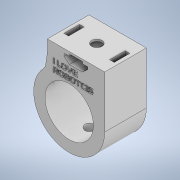
# Autodesk Inventor part: MotorBearingHolder
Saved by Autodesk Inventor 2020 (Build 240168000, 168)
## iProperties
Created: 2020-01-14
Part Number: MotorBearingHolder
Material: Generic
Document SubType Name: Modeling
Designer: yukin
Density: 1 g/cm^3
Appearance: Default
Author: yukin
Autodesk Inventor part; units mm, degrees
note: some values were not read from the file. Chosen so that the rebuilt part matches the saved one: direction of "Emboss1".
ref_plane "YZ Plane" through (0, 0, 0) normal (1, 0, 0) x (0, 1, 0)
sketch "Sketch1" plane through (0, 0, 0) normal (0, 0, 1) x (1, 0, 0)
  line L0 (-13.97, -12.7) -> (13.97, -12.7)
  line L1 (13.97, -12.7) -> (13.97, 12.7)
  line L2 (13.97, 12.7) -> (-13.97, 12.7)
  line L3 (-13.97, 12.7) -> (-13.97, -12.7)
  line L4 (-13.97, -12.7) -> (13.97, 12.7) construction
  line L5 (13.97, -12.7) -> (-13.97, 12.7) construction
  arc A0 (-13.97, -12.7) -> (13.97, -12.7) centre (0, -12.7) ccw
  circle A1 centre (-3.3455, -12.7) radius 11.811
  line L6 (0, -12.7) -> (-13.97, -12.7)
  line L7 (0, -12.7) -> (-6.985, -12.7)
  circle A2 centre (-3.3455, -12.7) radius 17.3155
  arc A3 (-20.6609, -12.7) -> (-13.97, 12.7) centre (-56.001, 10.1906) ccw
  point P0 (0, 0)
  point P1 (-15.1565, -0.038)
  dimension "d0" = 27.94
  dimension "d1" = 25.4
  dimension "d2" = 23.622
  constraints: 16 end point, 6 point on circle, 4 centre point, 3 midpoint, 2 parallel, 2 tangent, 1 coincident, 1 horizontal, 1 perpendicular
  measures "d0" distance of L1.end L2.end
  measures "d1" distance of L0.end L1.end
  measures "d2" diameter of A1
sketch "Sketch5" plane through (0, 0, 0) normal (0, 0, 1) x (1, 0, 0)
  line L0 (0, 12.7) -> (0, 6.35)
  line L1 (0, 12.7) -> (0, 9.525)
  line L2 (5.715, 7.3025) -> (-5.715, 7.3025)
  line L3 (-5.715, 7.3025) -> (-5.715, 11.7475)
  line L4 (-5.715, 11.7475) -> (5.715, 11.7475)
  line L5 (5.715, 11.7475) -> (5.715, 7.3025)
  line L6 (5.715, 7.3025) -> (-5.715, 11.7475) construction
  line L7 (-5.715, 7.3025) -> (5.715, 11.7475) construction
  line L8 (5.715, 11.7475) -> (3.175, 11.7475)
  line L9 (3.175, 11.7475) -> (3.175, 10.7597)
  line L10 (3.175, 10.7597) -> (5.715, 10.7597)
  line L11 (5.715, 10.7597) -> (5.715, 11.7475)
  line L12 (-5.715, 11.7475) -> (-3.2581, 11.7475)
  line L13 (-3.2581, 11.7475) -> (-3.2581, 10.792)
  line L14 (-3.2581, 10.792) -> (-5.715, 10.792)
  line L15 (-5.715, 10.792) -> (-5.715, 11.7475)
  line L16 (5.715, 9.525) -> (3.175, 7.3025)
  line L17 (-5.715, 9.525) -> (-3.175, 7.3025)
  point P0 (0, 0)
  point P1 (5.715, 10.7597)
  point P2 (-3.2581, 11.7475)
  point P3 (-5.715, 10.792)
  dimension "d5" = 4.445
  dimension "d6" = 11.43
  dimension "d7" = 2.54
  constraints: 36 end point, 6 parallel, 5 midpoint, 4 point on line, 3 horizontal, 3 perpendicular
  measures "d5" distance of L2.end L3.end
  measures "d6" distance of L2.start L2.end
  measures "d7" distance of L10.end L9.end
ref_plane "Work Plane4" through (-13.97, 12.7, 0) normal (0, 1, 0) x (1, 0, 0)
sketch "Sketch6" plane through (-13.97, 12.7, 0) normal (0, 1, 0) x (1, 0, 0)
  circle A0 centre (13.97, -10.16) radius 2.54
  dimension "d19" = 5.08
  constraints: 1 centre point
  measures "d19" diameter of A0
extrude "Extrusion7" add sketch "Sketch1" along normal blind 20.32 contours A1 A0 A2 A3 L3 | L3 A2 L0 A1 | A1 L0 A0 | A2 A3 L3 | L3 A3 L2 L1 A2 | A3 A2 picked at (12.0052, -13.7923)
extrude "Extrusion8" cut sketch "Sketch5" along normal blind 20.32 contours L4 L9 L10 L5 L16 L2 L0 | L0 L2 L17 L3 L14 L13 L4
extrude "Extrusion9" cut sketch "Sketch6" against normal blind 15.24
fillet "Fillet1" radius 3.175 1 edges at (-15.1565, -0.038, 10.16)
sketch "Sketch10" plane through (-13.97, 12.7, 0) normal (0, 1, 0) x (1, 0, 0)
  line L0 (13.97, 0) -> (13.97, -20.32)
  line L1 (0.0748, -20.32) -> (0.0748, 0) projected
  line L2 (0.0748, -10.16) -> (27.94, -10.16)
  line L3 (27.94, 0) -> (27.94, -20.32) projected
  line L4 (3.9773, -13.97) -> (1.6913, -13.97)
  line L5 (1.6913, -13.97) -> (1.6913, -6.35)
  line L6 (1.6913, -6.35) -> (3.9773, -6.35)
  line L7 (3.9773, -6.35) -> (3.9773, -13.97)
  line L8 (3.9773, -13.97) -> (1.6913, -6.35) construction
  line L9 (1.6913, -13.97) -> (3.9773, -6.35) construction
  line L10 (23.9627, -13.97) -> (26.2487, -13.97)
  line L11 (26.2487, -13.97) -> (26.2487, -6.35)
  line L12 (26.2487, -6.35) -> (23.9627, -6.35)
  line L13 (23.9627, -6.35) -> (23.9627, -13.97)
  point P0 (2.8343, -10.16)
  dimension "d32" = 2.286
  dimension "d33" = 7.62
  constraints: 24 end point, 4 midpoint, 4 symmetric about line, 2 parallel, 1 horizontal, 1 perpendicular, 1 point on line
  measures "d32" distance of L5.end L6.end
  measures "d33" distance of L6.end L4.start
extrude "Extrusion10" cut sketch "Sketch10" against normal blind 2.54
ref_plane "Work Plane5" through (-3.3455, -30.0155, 0) normal (0, 1, 0) x (-1, 0, 0)
sketch "Sketch11" plane through (-3.3455, -30.0155, 0) normal (0, 1, 0) x (-1, 0, 0)
  line L0 (-0.1705, 0) -> (-0.1705, 20.32) projected
  circle A0 centre (-0.1705, 10.16) radius 2.54
  point P0 (-3.3455, 0)
  dimension "d36" = 5.08
  constraints: 1 centre point, 1 midpoint
  measures "d36" diameter of A0
extrude "Extrusion11" cut sketch "Sketch11" along normal blind 15.24
sketch "Sketch12" plane through (0, 0, 20.32) normal (0, 0, 1) x (1, 0, 0)
  line L0 (-11.2307, 6.2995) -> (3.6868, 6.2995) construction
  line L1 (3.6868, 6.2995) -> (3.6868, 2.8789) construction
  line L2 (3.6868, 2.8789) -> (-11.2307, 2.8789) construction
  line L3 (-11.2307, 2.8789) -> (-11.2307, 6.2995) construction
  spline S0 degree 2 poles (-10.4241, 3.896) (-10.4282, 3.8288) (-10.526, 3.733) (-10.5972, 3.7371) knots 0 0 0 1 2 2 2
  line L4 (-10.5972, 3.7371) -> (-10.8702, 3.7534)
  spline S1 degree 2 poles (-10.8702, 3.7534) (-10.9374, 3.7575) (-11.0352, 3.8654) (-11.0352, 3.9327) knots 0 0 0 1 2 2 2
  line L5 (-11.0352, 3.9327) -> (-11.0698, 6.1345)
  spline S2 degree 2 poles (-11.0698, 6.1345) (-11.0698, 6.2058) (-10.968, 6.3016) (-10.8946, 6.2934) knots 0 0 0 1 2 2 2
  line L6 (-10.8946, 6.2934) -> (-10.5606, 6.2649)
  spline S3 degree 2 poles (-10.5606, 6.2649) (-10.4954, 6.2588) (-10.4017, 6.1549) (-10.4017, 6.1284) knots 0 0 0 1 2 2 2
  line L7 (-10.4017, 6.1284) -> (-10.4241, 3.896)
  spline S4 degree 2 poles (-9.1898, 6.0999) (-9.1898, 6.1671) (-9.0859, 6.2608) (-9.0146, 6.2547) knots 0 0 0 1 2 2 2
  line L8 (-9.0146, 6.2547) -> (-8.6805, 6.2242)
  spline S5 degree 2 poles (-8.6805, 6.2242) (-8.6194, 6.216) (-8.5196, 6.1182) (-8.5196, 6.0775) knots 0 0 0 1 2 2 2
  line L9 (-8.5196, 6.0775) -> (-8.5583, 4.3767)
  spline S6 degree 2 poles (-8.5583, 4.3767) (-8.5583, 4.3197) (-8.5135, 4.281) (-8.485, 4.283) knots 0 0 0 1 2 2 2
  line L10 (-8.485, 4.283) -> (-7.3912, 4.3217)
  spline S7 degree 2 poles (-7.3912, 4.3217) (-7.3403, 4.3217) (-7.2995, 4.281) knots 0 0 0 1 1 1
  spline S8 degree 2 poles (-7.2995, 4.281) (-7.2466, 4.2423) (-7.2466, 4.1791) knots 0 0 0 1 1 1
  line L11 (-7.2466, 4.1791) -> (-7.2812, 3.8899)
  spline S9 degree 2 poles (-7.2812, 3.8899) (-7.2771, 3.8288) (-7.3627, 3.7371) (-7.4278, 3.7371) knots 0 0 0 1 2 2 2
  line L12 (-7.4278, 3.7371) -> (-8.705, 3.7371)
  spline S10 degree 2 poles (-8.705, 3.7371) (-8.8027, 3.7371) (-8.9718, 3.8105) (-9.0961, 3.9347) (-9.1694, 4.1038) (-9.1694, 4.2015) knots 0 0 0 1 2 3 4 4 4
  line L13 (-9.1694, 4.2015) -> (-9.1898, 6.0999)
  spline S11 degree 2 poles (-4.6719, 5.6701) (-4.6577, 5.55) (-4.6353, 5.2383) (-4.6312, 4.9165) (-4.6434, 4.6008) (-4.6577, 4.4724) knots 0 0 0 1 2 3 4 4 4
  spline S12 degree 2 poles (-4.6577, 4.4724) (-4.6882, 4.1588) (-5.0039, 3.8288) (-5.3197, 3.7819) knots 0 0 0 1 2 2 2
  spline S13 degree 2 poles (-5.3197, 3.7819) (-5.4134, 3.7677) (-5.7006, 3.7493) (-6.0122, 3.7453) (-6.3218, 3.7555) (-6.44, 3.7677) knots 0 0 0 1 2 3 4 4 4
  spline S14 degree 2 poles (-6.44, 3.7677) (-6.6885, 3.786) (-7.051, 4.1241) (-7.0897, 4.395) knots 0 0 0 1 2 2 2
  spline S15 degree 2 poles (-7.0897, 4.395) (-7.1121, 4.5437) (-7.1305, 4.9002) (-7.1345, 5.2485) (-7.1203, 5.5683) (-7.104, 5.6783) knots 0 0 0 1 2 3 4 4 4
  spline S16 degree 2 poles (-7.104, 5.6783) (-7.0816, 5.8738) (-6.7883, 6.1569) (-6.5561, 6.1895) knots 0 0 0 1 2 2 2
  spline S17 degree 2 poles (-6.5561, 6.1895) (-6.4461, 6.1997) (-6.1141, 6.2262) (-5.7515, 6.2466) (-5.3971, 6.2527) (-5.2687, 6.2486) knots 0 0 0 1 2 3 4 4 4
  spline S18 degree 2 poles (-5.2687, 6.2486) (-4.9856, 6.2364) (-4.7045, 5.941) (-4.6719, 5.6701) knots 0 0 0 1 2 2 2
  spline S19 degree 2 poles (-5.34, 5.717) (-5.45, 5.7292) (-5.7332, 5.7333) (-6.0285, 5.7292) (-6.2933, 5.7068) (-6.387, 5.6925) knots 0 0 0 1 2 3 4 4 4
  spline S20 degree 2 poles (-6.387, 5.6925) (-6.4359, 5.6803) (-6.5051, 5.5988) (-6.5072, 5.5377) knots 0 0 0 1 2 2 2
  spline S21 degree 2 poles (-6.5072, 5.5377) (-6.5133, 5.44) (-6.5133, 5.1263) (-6.5031, 4.835) (-6.4848, 4.5478) (-6.4664, 4.4419) knots 0 0 0 1 2 3 4 4 4
  spline S22 degree 2 poles (-6.4664, 4.4419) (-6.4562, 4.3584) (-6.3666, 4.2749) (-6.2974, 4.2647) knots 0 0 0 1 2 2 2
  spline S23 degree 2 poles (-6.2974, 4.2647) (-6.2098, 4.2545) (-5.9531, 4.2463) (-5.6904, 4.2545) (-5.45, 4.2789) (-5.3665, 4.3013) knots 0 0 0 1 2 3 4 4 4
  spline S24 degree 2 poles (-5.3665, 4.3013) (-5.2952, 4.3197) (-5.2199, 4.4134) (-5.2137, 4.4724) knots 0 0 0 1 2 2 2
  spline S25 degree 2 poles (-5.2137, 4.4724) (-5.2015, 4.6048) (-5.1873, 4.9022) (-5.1832, 5.1976) (-5.1913, 5.4685) (-5.1995, 5.5683) knots 0 0 0 1 2 3 4 4 4
  spline S26 degree 2 poles (-5.1995, 5.5683) (-5.2056, 5.6274) (-5.283, 5.7109) (-5.34, 5.717) knots 0 0 0 1 2 2 2
  spline S27 degree 2 poles (-2.3417, 6.1794) (-2.3112, 6.2343) (-2.1829, 6.2792) (-2.1238, 6.2506) knots 0 0 0 1 2 2 2
  line L14 (-2.1238, 6.2506) -> (-1.8508, 6.1284)
  spline S28 degree 2 poles (-1.8508, 6.1284) (-1.7857, 6.102) (-1.7531, 5.9818) (-1.7714, 5.939) knots 0 0 0 1 2 2 2
  line L15 (-1.7714, 5.939) -> (-2.6147, 4.0264)
  spline S29 degree 2 poles (-2.6147, 4.0264) (-2.6839, 3.8797) (-2.9589, 3.733) (-3.2563, 3.733) (-3.5252, 3.8777) (-3.5965, 4.0223) knots 0 0 0 1 2 3 4 4 4
  line L16 (-3.5965, 4.0223) -> (-4.4377, 5.939)
  spline S30 degree 2 poles (-4.4377, 5.939) (-4.456, 5.9818) (-4.4275, 6.0999) (-4.3521, 6.1325) knots 0 0 0 1 2 2 2
  line L17 (-4.3521, 6.1325) -> (-4.0894, 6.2486)
  spline S31 degree 2 poles (-4.0894, 6.2486) (-4.0324, 6.2792) (-3.8979, 6.2343) (-3.8714, 6.1753) knots 0 0 0 1 2 2 2
  line L18 (-3.8714, 6.1753) -> (-3.1259, 4.3869)
  spline S32 degree 2 poles (-3.1259, 4.3869) (-3.1219, 4.3787) (-3.0893, 4.3787) (-3.0832, 4.3869) knots 0 0 0 1 2 2 2
  line L19 (-3.0832, 4.3869) -> (-2.3417, 6.1794)
  line L20 (-0.9689, 4.7433) -> (-0.9648, 4.393)
  spline S33 degree 2 poles (-0.9648, 4.393) (-0.9628, 4.3604) (-0.922, 4.3197) (-0.8935, 4.3176) knots 0 0 0 1 2 2 2
  line L21 (-0.8935, 4.3176) -> (0.6443, 4.2463)
  spline S34 degree 2 poles (0.6443, 4.2463) (0.7177, 4.2463) (0.7645, 4.2076) knots 0 0 0 1 1 1
  spline S35 degree 2 poles (0.7645, 4.2076) (0.8175, 4.1649) (0.8175, 4.118) knots 0 0 0 1 1 1
  line L22 (0.8175, 4.118) -> (0.8093, 3.9449)
  spline S36 degree 2 poles (0.8093, 3.9449) (0.8093, 3.8736) (0.7279, 3.7819) (0.6586, 3.7819) knots 0 0 0 1 2 2 2
  line L23 (0.6586, 3.7819) -> (-1.087, 3.7636)
  spline S37 degree 2 poles (-1.087, 3.7636) (-1.2866, 3.7636) (-1.4292, 3.894) knots 0 0 0 1 1 1
  spline S38 degree 2 poles (-1.4292, 3.894) (-1.5718, 4.0365) (-1.5718, 4.2362) knots 0 0 0 1 1 1
  line L24 (-1.5718, 4.2362) -> (-1.5494, 5.7822)
  spline S39 degree 2 poles (-1.5494, 5.7822) (-1.5494, 5.8759) (-1.4801, 6.0429) (-1.364, 6.1631) (-1.197, 6.2425) (-1.0646, 6.2425) knots 0 0 0 1 2 3 4 4 4
  line L25 (-1.0646, 6.2425) -> (0.5975, 6.269)
  spline S40 degree 2 poles (0.5975, 6.269) (0.6647, 6.2751) (0.7116, 6.2282) knots 0 0 0 1 1 1
  spline S41 degree 2 poles (0.7116, 6.2282) (0.7523, 6.1956) (0.7625, 6.1325) knots 0 0 0 1 1 1
  line L26 (0.7625, 6.1325) -> (0.7706, 5.8535)
  spline S42 degree 2 poles (0.7706, 5.8535) (0.7747, 5.7903) (0.6892, 5.6986) (0.6219, 5.6986) knots 0 0 0 1 2 2 2
  line L27 (0.6219, 5.6986) -> (-0.9118, 5.7598)
  spline S43 degree 2 poles (-0.9118, 5.7598) (-0.9404, 5.7598) (-0.9607, 5.7353) knots 0 0 0 1 1 1
  spline S44 degree 2 poles (-0.9607, 5.7353) (-0.9811, 5.7211) (-0.9811, 5.6538) knots 0 0 0 1 1 1
  line L28 (-0.9811, 5.6538) -> (-0.977, 5.2628)
  line L29 (-0.977, 5.2628) -> (0.4529, 5.334)
  spline S45 degree 2 poles (0.4529, 5.334) (0.5201, 5.3422) (0.5649, 5.2953) knots 0 0 0 1 1 1
  spline S46 degree 2 poles (0.5649, 5.2953) (0.5873, 5.2811) (0.6138, 5.2261) (0.6179, 5.2016) knots 0 0 0 1 2 2 2
  line L30 (0.6179, 5.2016) -> (0.626, 4.888)
  spline S47 degree 2 poles (0.626, 4.888) (0.6301, 4.8248) (0.5445, 4.7291) (0.4773, 4.7291) knots 0 0 0 1 2 2 2
  line L31 (0.4773, 4.7291) -> (-0.9689, 4.7433)
  spline S48 degree 2 poles (-8.6215, 2.1971) (-8.6133, 2.1442) (-8.6011, 1.9853) (-8.6011, 1.8346) (-8.6092, 1.6736) (-8.6133, 1.6329) knots 0 0 0 1 2 3 4 4 4
  spline S49 degree 2 poles (-8.6133, 1.6329) (-8.6439, 1.417) (-8.8842, 1.1318) (-9.0574, 1.0952) knots 0 0 0 1 2 2 2
  line L32 (-9.0574, 1.0952) -> (-8.6846, 0.4922)
  spline S50 degree 2 poles (-8.6846, 0.4922) (-8.65, 0.4332) (-8.6948, 0.2987) (-8.7498, 0.2743) knots 0 0 0 1 2 2 2
  line L33 (-8.7498, 0.2743) -> (-9.0675, 0.1358)
  spline S51 degree 2 poles (-9.0675, 0.1358) (-9.1286, 0.1175) (-9.257, 0.1521) (-9.2814, 0.1949) knots 0 0 0 1 2 2 2
  line L34 (-9.2814, 0.1949) -> (-9.7173, 1.0341)
  spline S52 degree 2 poles (-9.7173, 1.0341) (-9.8925, 1.0259) (-10.2999, 1.0259) (-10.4506, 1.0341) knots 0 0 0 1 2 2 2
  line L35 (-10.4506, 1.0341) -> (-10.4424, 0.2886)
  spline S53 degree 2 poles (-10.4424, 0.2886) (-10.4424, 0.26) (-10.53, 0.1663) (-10.5911, 0.1623) knots 0 0 0 1 2 2 2
  line L36 (-10.5911, 0.1623) -> (-10.8926, 0.1358)
  spline S54 degree 2 poles (-10.8926, 0.1358) (-10.9618, 0.1276) (-11.0596, 0.2193) (-11.0555, 0.2865) knots 0 0 0 1 2 2 2
  line L37 (-11.0555, 0.2865) -> (-11.0291, 2.3173)
  spline S55 degree 2 poles (-11.0291, 2.3173) (-11.0291, 2.4375) (-10.862, 2.5801) (-10.7541, 2.5964) knots 0 0 0 1 2 2 2
  spline S56 degree 2 poles (-10.7541, 2.5964) (-10.3528, 2.6493) (-9.5523, 2.6717) (-9.206, 2.6575) knots 0 0 0 1 2 2 2
  spline S57 degree 2 poles (-9.206, 2.6575) (-8.9759, 2.6412) (-8.6683, 2.3845) (-8.6215, 2.1971) knots 0 0 0 1 2 2 2
  spline S58 degree 2 poles (-10.4567, 1.527) (-10.3569, 1.5209) (-10.0188, 1.5168) (-9.6766, 1.5249) (-9.369, 1.5433) (-9.2692, 1.5616) knots 0 0 0 1 2 3 4 4 4
  spline S59 degree 2 poles (-9.2692, 1.5616) (-9.1836, 1.5738) (-9.1572, 1.6716) knots 0 0 0 1 1 1
  spline S60 degree 2 poles (-9.1572, 1.6716) (-9.1551, 1.6838) (-9.1429, 1.7979) (-9.1388, 1.9221) (-9.1388, 2.0301) (-9.1388, 2.0423) knots 0 0 0 1 2 3 4 4 4
  spline S61 degree 2 poles (-9.1388, 2.0423) (-9.1449, 2.0892) (-9.1959, 2.1462) (-9.2468, 2.1523) knots 0 0 0 1 2 2 2
  spline S62 degree 2 poles (-9.2468, 2.1523) (-9.3547, 2.1605) (-9.6358, 2.1645) (-9.9393, 2.1564) (-10.251, 2.1381) (-10.3976, 2.1258) knots 0 0 0 1 2 3 4 4 4
  spline S63 degree 2 poles (-10.3976, 2.1258) (-10.4241, 2.1238) (-10.4628, 2.0851) (-10.4628, 2.0199) knots 0 0 0 1 2 2 2
  line L38 (-10.4628, 2.0199) -> (-10.4567, 1.527)
  spline S64 degree 2 poles (-5.9022, 2.0769) (-5.888, 1.9568) (-5.8656, 1.6451) (-5.8615, 1.3233) (-5.8737, 1.0076) (-5.888, 0.8793) knots 0 0 0 1 2 3 4 4 4
  spline S65 degree 2 poles (-5.888, 0.8793) (-5.9185, 0.5656) (-6.2342, 0.2356) (-6.5499, 0.1887) knots 0 0 0 1 2 2 2
  spline S66 degree 2 poles (-6.5499, 0.1887) (-6.6436, 0.1745) (-6.9308, 0.1562) (-7.2425, 0.1521) (-7.5521, 0.1623) (-7.6702, 0.1745) knots 0 0 0 1 2 3 4 4 4
  spline S67 degree 2 poles (-7.6702, 0.1745) (-7.9187, 0.1928) (-8.2813, 0.5309) (-8.32, 0.8019) knots 0 0 0 1 2 2 2
  spline S68 degree 2 poles (-8.32, 0.8019) (-8.3424, 0.9505) (-8.3607, 1.307) (-8.3648, 1.6553) (-8.3506, 1.9751) (-8.3343, 2.0851) knots 0 0 0 1 2 3 4 4 4
  spline S69 degree 2 poles (-8.3343, 2.0851) (-8.3119, 2.2806) (-8.0185, 2.5638) (-7.7863, 2.5964) knots 0 0 0 1 2 2 2
  spline S70 degree 2 poles (-7.7863, 2.5964) (-7.6763, 2.6065) (-7.3443, 2.633) (-6.9818, 2.6534) (-6.6273, 2.6595) (-6.499, 2.6554) knots 0 0 0 1 2 3 4 4 4
  spline S71 degree 2 poles (-6.499, 2.6554) (-6.2159, 2.6432) (-5.9348, 2.3478) (-5.9022, 2.0769) knots 0 0 0 1 2 2 2
  spline S72 degree 2 poles (-6.5703, 2.1238) (-6.6803, 2.136) (-6.9634, 2.1401) (-7.2588, 2.136) (-7.5236, 2.1136) (-7.6173, 2.0993) knots 0 0 0 1 2 3 4 4 4
  spline S73 degree 2 poles (-7.6173, 2.0993) (-7.6662, 2.0871) (-7.7354, 2.0057) (-7.7375, 1.9445) knots 0 0 0 1 2 2 2
  spline S74 degree 2 poles (-7.7375, 1.9445) (-7.7436, 1.8468) (-7.7436, 1.5331) (-7.7334, 1.2418) (-7.715, 0.9546) (-7.6967, 0.8487) knots 0 0 0 1 2 3 4 4 4
  spline S75 degree 2 poles (-7.6967, 0.8487) (-7.6865, 0.7652) (-7.5969, 0.6817) (-7.5277, 0.6715) knots 0 0 0 1 2 2 2
  spline S76 degree 2 poles (-7.5277, 0.6715) (-7.4401, 0.6613) (-7.1834, 0.6532) (-6.9207, 0.6613) (-6.6803, 0.6857) (-6.5968, 0.7082) knots 0 0 0 1 2 3 4 4 4
  spline S77 degree 2 poles (-6.5968, 0.7082) (-6.5255, 0.7265) (-6.4501, 0.8202) (-6.444, 0.8793) knots 0 0 0 1 2 2 2
  spline S78 degree 2 poles (-6.444, 0.8793) (-6.4318, 1.0117) (-6.4175, 1.309) (-6.4135, 1.6044) (-6.4216, 1.8753) (-6.4298, 1.9751) knots 0 0 0 1 2 3 4 4 4
  spline S79 degree 2 poles (-6.4298, 1.9751) (-6.4359, 2.0342) (-6.5133, 2.1177) (-6.5703, 2.1238) knots 0 0 0 1 2 2 2
  spline S80 degree 2 poles (-3.2706, 2.1951) (-3.2563, 2.1258) (-3.2522, 1.8977) (-3.2604, 1.8183) knots 0 0 0 1 2 2 2
  spline S81 degree 2 poles (-3.2604, 1.8183) (-3.2848, 1.6207) (-3.3826, 1.5127) knots 0 0 0 1 1 1
  spline S82 degree 2 poles (-3.3826, 1.5127) (-3.3011, 1.47) (-3.1687, 1.2826) (-3.1483, 1.1787) knots 0 0 0 1 2 2 2
  spline S83 degree 2 poles (-3.1483, 1.1787) (-3.1259, 1.0789) (-3.1219, 0.8406) (-3.1341, 0.755) knots 0 0 0 1 2 2 2
  spline S84 degree 2 poles (-3.1341, 0.755) (-3.1646, 0.5167) (-3.46, 0.2213) (-3.7064, 0.1969) knots 0 0 0 1 2 2 2
  spline S85 degree 2 poles (-3.7064, 0.1969) (-3.8653, 0.1786) (-4.2625, 0.1602) (-4.6842, 0.1521) (-5.1038, 0.1643) (-5.2891, 0.1745) knots 0 0 0 1 2 3 4 4 4
  spline S86 degree 2 poles (-5.2891, 0.1745) (-5.4358, 0.1867) (-5.5987, 0.366) (-5.5987, 0.5045) knots 0 0 0 1 2 2 2
  line L39 (-5.5987, 0.5045) -> (-5.5722, 2.2908)
  spline S87 degree 2 poles (-5.5722, 2.2908) (-5.5722, 2.3947) (-5.4378, 2.5821) (-5.3176, 2.6065) knots 0 0 0 1 2 2 2
  spline S88 degree 2 poles (-5.3176, 2.6065) (-5.118, 2.633) (-4.7392, 2.6717) (-4.3786, 2.686) (-4.0324, 2.6819) (-3.8572, 2.6717) knots 0 0 0 1 2 3 4 4 4
  spline S89 degree 2 poles (-3.8572, 2.6717) (-3.625, 2.6554) (-3.3031, 2.4069) (-3.2706, 2.1951) knots 0 0 0 1 2 2 2
  spline S90 degree 2 poles (-4.9897, 0.7143) (-4.9897, 0.6878) (-4.951, 0.6491) (-4.9225, 0.647) knots 0 0 0 1 2 2 2
  spline S91 degree 2 poles (-4.9225, 0.647) (-4.7962, 0.643) (-4.4764, 0.647) (-4.1607, 0.6572) (-3.8837, 0.6756) (-3.7961, 0.6898) knots 0 0 0 1 2 3 4 4 4
  spline S92 degree 2 poles (-3.7961, 0.6898) (-3.7044, 0.702) (-3.6779, 0.7998) knots 0 0 0 1 1 1
  spline S93 degree 2 poles (-3.6779, 0.7998) (-3.6739, 0.81) (-3.6637, 0.8935) (-3.6596, 0.975) (-3.6596, 1.0524) (-3.6596, 1.0626) knots 0 0 0 1 2 3 4 4 4
  spline S94 degree 2 poles (-3.6596, 1.0626) (-3.6657, 1.1074) (-3.7146, 1.1644) (-3.7676, 1.1705) knots 0 0 0 1 2 2 2
  spline S95 degree 2 poles (-3.7676, 1.1705) (-3.8857, 1.1827) (-4.1933, 1.1827) (-4.5314, 1.1705) (-4.8736, 1.1522) (-4.9938, 1.14) knots 0 0 0 1 2 3 4 4 4
  line L40 (-4.9938, 1.14) -> (-4.9897, 0.7143)
  spline S96 degree 2 poles (-4.9999, 1.6696) (-4.9041, 1.6655) (-4.6006, 1.6614) (-4.2971, 1.6675) (-4.0242, 1.6899) (-3.9264, 1.7042) knots 0 0 0 1 2 3 4 4 4
  spline S97 degree 2 poles (-3.9264, 1.7042) (-3.8735, 1.7123) (-3.8246, 1.7612) (-3.8063, 1.806) knots 0 0 0 1 2 2 2
  spline S98 degree 2 poles (-3.8063, 1.806) (-3.8022, 1.8203) (-3.794, 1.8916) (-3.792, 1.9771) (-3.792, 2.0545) (-3.792, 2.0708) knots 0 0 0 1 2 3 4 4 4
  spline S99 degree 2 poles (-3.792, 2.0708) (-3.794, 2.1136) (-3.8551, 2.1645) (-3.8959, 2.1666) knots 0 0 0 1 2 2 2
  spline S100 degree 2 poles (-3.8959, 2.1666) (-4.1179, 2.1747) (-4.678, 2.1625) (-4.9449, 2.1401) knots 0 0 0 1 2 2 2
  spline S101 degree 2 poles (-4.9449, 2.1401) (-4.9693, 2.1381) (-5.0019, 2.0993) (-5.0019, 2.0362) knots 0 0 0 1 2 2 2
  line L41 (-5.0019, 2.0362) -> (-4.9999, 1.6696)
  spline S102 degree 2 poles (-0.425, 2.0769) (-0.4108, 1.9568) (-0.3884, 1.6451) (-0.3843, 1.3233) (-0.3965, 1.0076) (-0.4108, 0.8793) knots 0 0 0 1 2 3 4 4 4
  spline S103 degree 2 poles (-0.4108, 0.8793) (-0.4413, 0.5656) (-0.757, 0.2356) (-1.0728, 0.1887) knots 0 0 0 1 2 2 2
  spline S104 degree 2 poles (-1.0728, 0.1887) (-1.1664, 0.1745) (-1.4537, 0.1562) (-1.7653, 0.1521) (-2.0749, 0.1623) (-2.193, 0.1745) knots 0 0 0 1 2 3 4 4 4
  spline S105 degree 2 poles (-2.193, 0.1745) (-2.4415, 0.1928) (-2.8041, 0.5309) (-2.8428, 0.8019) knots 0 0 0 1 2 2 2
  spline S106 degree 2 poles (-2.8428, 0.8019) (-2.8652, 0.9505) (-2.8835, 1.307) (-2.8876, 1.6553) (-2.8734, 1.9751) (-2.8571, 2.0851) knots 0 0 0 1 2 3 4 4 4
  spline S107 degree 2 poles (-2.8571, 2.0851) (-2.8347, 2.2806) (-2.5413, 2.5638) (-2.3091, 2.5964) knots 0 0 0 1 2 2 2
  spline S108 degree 2 poles (-2.3091, 2.5964) (-2.1992, 2.6065) (-1.8671, 2.633) (-1.5046, 2.6534) (-1.1502, 2.6595) (-1.0218, 2.6554) knots 0 0 0 1 2 3 4 4 4
  spline S109 degree 2 poles (-1.0218, 2.6554) (-0.7387, 2.6432) (-0.4576, 2.3478) (-0.425, 2.0769) knots 0 0 0 1 2 2 2
  spline S110 degree 2 poles (-1.0931, 2.1238) (-1.2031, 2.136) (-1.4862, 2.1401) (-1.7816, 2.136) (-2.0464, 2.1136) (-2.1401, 2.0993) knots 0 0 0 1 2 3 4 4 4
  spline S111 degree 2 poles (-2.1401, 2.0993) (-2.189, 2.0871) (-2.2582, 2.0057) (-2.2603, 1.9445) knots 0 0 0 1 2 2 2
  spline S112 degree 2 poles (-2.2603, 1.9445) (-2.2664, 1.8468) (-2.2664, 1.5331) (-2.2562, 1.2418) (-2.2379, 0.9546) (-2.2195, 0.8487) knots 0 0 0 1 2 3 4 4 4
  spline S113 degree 2 poles (-2.2195, 0.8487) (-2.2093, 0.7652) (-2.1197, 0.6817) (-2.0505, 0.6715) knots 0 0 0 1 2 2 2
  spline S114 degree 2 poles (-2.0505, 0.6715) (-1.9629, 0.6613) (-1.7062, 0.6532) (-1.4435, 0.6613) (-1.2031, 0.6857) (-1.1196, 0.7082) knots 0 0 0 1 2 3 4 4 4
  spline S115 degree 2 poles (-1.1196, 0.7082) (-1.0483, 0.7265) (-0.9729, 0.8202) (-0.9668, 0.8793) knots 0 0 0 1 2 2 2
  spline S116 degree 2 poles (-0.9668, 0.8793) (-0.9546, 1.0117) (-0.9404, 1.309) (-0.9363, 1.6044) (-0.9444, 1.8753) (-0.9526, 1.9751) knots 0 0 0 1 2 3 4 4 4
  spline S117 degree 2 poles (-0.9526, 1.9751) (-0.9587, 2.0342) (-1.0361, 2.1177) (-1.0931, 2.1238) knots 0 0 0 1 2 2 2
  line L42 (1.2961, 2.1136) -> (1.3186, 0.2886)
  spline S118 degree 2 poles (1.3186, 0.2886) (1.3186, 0.2641) (1.231, 0.1725) (1.1699, 0.1623) knots 0 0 0 1 2 2 2
  line L43 (1.1699, 0.1623) -> (0.8664, 0.1358)
  spline S119 degree 2 poles (0.8664, 0.1358) (0.793, 0.1317) (0.7014, 0.2173) (0.7014, 0.2865) knots 0 0 0 1 2 2 2
  line L44 (0.7014, 0.2865) -> (0.7238, 2.1136)
  line L45 (0.7238, 2.1136) -> (-0.0767, 2.1136)
  spline S120 degree 2 poles (-0.0767, 2.1136) (-0.1399, 2.1136) (-0.1908, 2.1564) knots 0 0 0 1 1 1
  spline S121 degree 2 poles (-0.1908, 2.1564) (-0.203, 2.1706) (-0.2336, 2.2256) (-0.2315, 2.2623) knots 0 0 0 1 2 2 2
  line L46 (-0.2315, 2.2623) -> (-0.2274, 2.4314)
  spline S122 degree 2 poles (-0.2274, 2.4314) (-0.2234, 2.4884) (-0.1419, 2.578) (-0.0706, 2.578) knots 0 0 0 1 2 2 2
  line L47 (-0.0706, 2.578) -> (2.0905, 2.686)
  spline S123 degree 2 poles (2.0905, 2.686) (2.1394, 2.686) (2.1944, 2.6412) knots 0 0 0 1 1 1
  spline S124 degree 2 poles (2.1944, 2.6412) (2.2392, 2.5964) (2.2392, 2.5271) knots 0 0 0 1 1 1
  line L48 (2.2392, 2.5271) -> (2.2494, 2.2684)
  spline S125 degree 2 poles (2.2494, 2.2684) (2.2555, 2.2053) (2.1679, 2.1136) (2.1028, 2.1136) knots 0 0 0 1 2 2 2
  line L49 (2.1028, 2.1136) -> (1.2961, 2.1136)
  spline S126 degree 2 poles (4.5715, 0.812) (4.6387, 0.8283) (4.7405, 0.7611) (4.7446, 0.7061) knots 0 0 0 1 2 2 2
  line L50 (4.7446, 0.7061) -> (4.767, 0.4006)
  spline S127 degree 2 poles (4.767, 0.4006) (4.7711, 0.3354) (4.6815, 0.256) (4.6366, 0.2478) knots 0 0 0 1 2 2 2
  spline S128 degree 2 poles (4.6366, 0.2478) (4.2211, 0.1826) (3.4064, 0.1867) (3.0153, 0.2356) knots 0 0 0 1 2 2 2
  spline S129 degree 2 poles (3.0153, 0.2356) (2.4694, 0.2987) (2.4368, 0.7978) knots 0 0 0 1 1 1
  spline S130 degree 2 poles (2.4368, 0.7978) (2.4185, 1.1216) (2.4266, 1.749) (2.4572, 2.0484) knots 0 0 0 1 2 2 2
  spline S131 degree 2 poles (2.4572, 2.0484) (2.4674, 2.1462) (2.559, 2.3417) (2.7016, 2.4925) (2.8931, 2.5882) (3.0071, 2.6004) knots 0 0 0 1 2 3 4 4 4
  spline S132 degree 2 poles (3.0071, 2.6004) (3.3575, 2.6371) (4.1396, 2.6534) (4.5287, 2.6269) knots 0 0 0 1 2 2 2
  spline S133 degree 2 poles (4.5287, 2.6269) (4.5837, 2.6208) (4.6774, 2.5536) (4.6815, 2.4884) knots 0 0 0 1 2 2 2
  line L51 (4.6815, 2.4884) -> (4.6916, 2.2134)
  spline S134 degree 2 poles (4.6916, 2.2134) (4.6978, 2.1503) (4.6102, 2.0505) (4.5389, 2.0545) knots 0 0 0 1 2 2 2
  spline S135 degree 2 poles (4.5389, 2.0545) (4.1885, 2.0912) (3.5184, 2.1218) (3.1986, 2.1218) knots 0 0 0 1 2 2 2
  spline S136 degree 2 poles (3.1986, 2.1218) (3.1395, 2.1218) (3.0295, 2.0118) (3.0234, 1.9405) knots 0 0 0 1 2 2 2
  spline S137 degree 2 poles (3.0234, 1.9405) (3.0051, 1.7001) (3.0092, 1.1481) (3.0377, 0.9139) knots 0 0 0 1 2 2 2
  spline S138 degree 2 poles (3.0377, 0.9139) (3.0397, 0.8894) (3.0805, 0.8263) (3.1334, 0.7733) (3.1966, 0.7387) (3.2251, 0.7367) knots 0 0 0 1 2 3 4 4 4
  spline S139 degree 2 poles (3.2251, 0.7367) (3.4125, 0.7183) (3.7363, 0.7061) (4.05, 0.7285) (4.3943, 0.7794) (4.5715, 0.812) knots 0 0 0 1 2 3 4 4 4
  spline S140 degree 2 poles (5.6531, 0.3028) (5.649, 0.2356) (5.5512, 0.1399) (5.4799, 0.1439) knots 0 0 0 1 2 2 2
  line L52 (5.4799, 0.1439) -> (5.207, 0.1602)
  spline S141 degree 2 poles (5.207, 0.1602) (5.1398, 0.1643) (5.042, 0.2723) (5.042, 0.3395) knots 0 0 0 1 2 2 2
  line L53 (5.042, 0.3395) -> (5.0074, 2.5414)
  spline S142 degree 2 poles (5.0074, 2.5414) (5.0074, 2.6126) (5.1092, 2.7084) (5.1825, 2.7002) knots 0 0 0 1 2 2 2
  line L54 (5.1825, 2.7002) -> (5.5166, 2.6717)
  spline S143 degree 2 poles (5.5166, 2.6717) (5.5818, 2.6656) (5.6755, 2.5617) (5.6755, 2.5352) knots 0 0 0 1 2 2 2
  line L55 (5.6755, 2.5352) -> (5.6531, 0.3028)
  spline S144 degree 2 poles (7.6472, 0.6837) (7.7653, 0.6837) (7.7694, 0.812) knots 0 0 0 1 1 1
  spline S145 degree 2 poles (7.7694, 0.812) (7.7694, 0.8181) (7.7694, 0.8691) (7.7653, 0.9241) (7.7653, 0.9791) (7.7653, 0.9852) knots 0 0 0 1 2 3 4 4 4
  spline S146 degree 2 poles (7.7653, 0.9852) (7.747, 1.0972) (7.6349, 1.1094) knots 0 0 0 1 1 1
  spline S147 degree 2 poles (7.6349, 1.1094) (7.3416, 1.14) (6.7245, 1.1583) (6.4332, 1.1889) knots 0 0 0 1 2 2 2
  spline S148 degree 2 poles (6.4332, 1.1889) (6.1928, 1.2113) (5.9301, 1.5066) (5.9301, 1.7429) knots 0 0 0 1 2 2 2
  spline S149 degree 2 poles (5.9301, 1.7429) (5.9301, 1.7775) (5.9301, 1.8773) (5.9382, 1.9792) (5.9423, 2.079) (5.9484, 2.1095) knots 0 0 0 1 2 3 4 4 4
  spline S150 degree 2 poles (5.9484, 2.1095) (5.9851, 2.3316) (6.2254, 2.6086) (6.4474, 2.6289) knots 0 0 0 1 2 2 2
  spline S151 degree 2 poles (6.4474, 2.6289) (6.8507, 2.6738) (7.7348, 2.688) (8.1177, 2.6595) knots 0 0 0 1 2 2 2
  spline S152 degree 2 poles (8.1177, 2.6595) (8.1747, 2.6595) (8.2236, 2.6228) knots 0 0 0 1 1 1
  spline S153 degree 2 poles (8.2236, 2.6228) (8.2806, 2.578) (8.2806, 2.4965) knots 0 0 0 1 1 1
  line L56 (8.2806, 2.4965) -> (8.2868, 2.2419)
  spline S154 degree 2 poles (8.2868, 2.2419) (8.2908, 2.1788) (8.2053, 2.0871) (8.136, 2.0871) knots 0 0 0 1 2 2 2
  spline S155 degree 2 poles (8.136, 2.0871) (7.7836, 2.1197) (6.9933, 2.1503) (6.643, 2.1503) knots 0 0 0 1 2 2 2
  spline S156 degree 2 poles (6.643, 2.1503) (6.5208, 2.1503) (6.5208, 2.0219) knots 0 0 0 1 1 1
  spline S157 degree 2 poles (6.5208, 2.0219) (6.5167, 2.0016) (6.5208, 1.8895) (6.5248, 1.8671) knots 0 0 0 1 2 2 2
  spline S158 degree 2 poles (6.5248, 1.8671) (6.5411, 1.7531) (6.6511, 1.7429) knots 0 0 0 1 1 1
  spline S159 degree 2 poles (6.6511, 1.7429) (6.7957, 1.7266) (7.0972, 1.7083) (7.4089, 1.694) (7.7144, 1.6777) (7.861, 1.6635) knots 0 0 0 1 2 3 4 4 4
  spline S160 degree 2 poles (7.861, 1.6635) (8.0953, 1.6349) (8.356, 1.3437) (8.356, 1.1115) knots 0 0 0 1 2 2 2
  spline S161 degree 2 poles (8.356, 1.1115) (8.356, 1.0768) (8.356, 0.9811) (8.3479, 0.8609) (8.3397, 0.755) (8.3356, 0.7183) knots 0 0 0 1 2 3 4 4 4
  spline S162 degree 2 poles (8.3356, 0.7183) (8.301, 0.5024) (8.0627, 0.2234) (7.8427, 0.203) knots 0 0 0 1 2 2 2
  spline S163 degree 2 poles (7.8427, 0.203) (7.639, 0.1806) (7.1889, 0.1541) (6.7326, 0.148) (6.2906, 0.1582) (6.1012, 0.1745) knots 0 0 0 1 2 3 4 4 4
  spline S164 degree 2 poles (6.1012, 0.1745) (6.034, 0.1745) (5.9932, 0.2132) knots 0 0 0 1 1 1
  spline S165 degree 2 poles (5.9932, 0.2132) (5.9423, 0.2519) (5.9423, 0.315) knots 0 0 0 1 1 1
  line L57 (5.9423, 0.315) -> (5.9301, 0.5961)
  spline S166 degree 2 poles (5.9301, 0.5961) (5.9301, 0.6572) (6.0156, 0.7469) (6.0788, 0.7469) knots 0 0 0 1 2 2 2
  spline S167 degree 2 poles (6.0788, 0.7469) (6.2621, 0.7265) (6.6613, 0.7041) (7.0728, 0.6898) (7.4394, 0.6837) (7.6472, 0.6837) knots 0 0 0 1 2 3 4 4 4
  point P0 (0, 0)
  constraints: 2 other
emboss "Emboss1" sketch "Sketch12" operation cut depth 2.54 direction (0, 0, -1)
body "Solid2"
